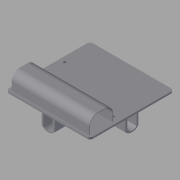
# Autodesk Inventor part: finalbody
Saved by Autodesk Inventor 2015 (Build 190159000, 159)
## iProperties
Created: 2015-11-09
Part Number: finalbody
Material: Generic
Document SubType Name: Modeling
Designer: Ross
Density: 1 g/cm^3
Appearance: Default
Author: Ross
Autodesk Inventor part; units mm, degrees
ref_plane "YZ Plane" through (0, 0, 0) normal (1, 0, 0) x (0, 1, 0)
ref_plane "XZ Plane" through (0, 0, 0) normal (0, 1, 0) x (-1, 0, 0)
sketch "Sketch1" plane through (0, 0, 0) normal (0, 1, 0) x (-1, 0, 0)
  line L0 (70, 0) -> (70, -70)
  line L1 (70, -70) -> (0, -70)
  line L2 (-70, 0) -> (-70, 70)
  line L3 (-70, 70) -> (0, 70)
  line L4 (0, 70) -> (70, 70)
  line L5 (70, 70) -> (70, 0)
  line L6 (0, -70) -> (-70, -70)
  line L7 (-70, -70) -> (-70, 0)
  point P0 (0, 0)
  constraints: 16 end point, 4 perpendicular, 2 point on line, 1 vertical
extrude "Extrusion1" add sketch "Sketch1" along normal blind 3
fillet "Fillet1" radius 5 3 edges at (70, 1.5, 70) (70, 1.5, -70) (-70, 1.5, 70)
fillet "Fillet2" radius 5 1 edges at (-70, 1.5, -70)
ref_plane "Work Plane1" through (65, 0, 65) normal (1, 0, 0) x (0, 0, -1)
sketch "Sketch5" plane through (65, 0, 65) normal (1, 0, 0) x (0, 0, -1)
  line L0 (0, 3) -> (0, 15.5)
  arc A0 (12.5, 28) -> (0, 15.5) centre (12.5, 15.5) ccw
  line L1 (12.5, 28) -> (25, 28)
  arc A1 (37.5, 15.5) -> (25, 28) centre (25, 15.5) ccw
  line L2 (37.5, 15.5) -> (37.5, 3)
  line L3 (0, 3) -> (130, 3) projected
  line L4 (0, 3) -> (-1, 3)
  line L5 (-5, 3) -> (0, 3) projected
  line L6 (-1, 3) -> (-1, 15.5)
  arc A2 (12.5, 29) -> (-1, 15.5) centre (12.5, 15.5) ccw
  line L7 (12.5, 29) -> (25, 29)
  arc A3 (38.5, 15.5) -> (25, 29) centre (25, 15.5) ccw
  line L8 (38.5, 15.5) -> (38.5, 3)
  line L9 (38.5, 3) -> (37.5, 3)
  line L10 (0, 3) -> (-1, 3)
  line L11 (0, 0) -> (0, 3) projected
  point P0 (65, 0)
  dimension "d9" = 12.5
  dimension "d11" = 12.5
  dimension "d12" = 1
  constraints: 18 end point, 8 point on circle, 4 centre point, 3 perpendicular, 3 point on line, 2 coincident, 2 vertical, 1 collinear, 1 horizontal, 1 parallel
  measures "d9" distance of L0.start L0.end
  measures "d11" distance of L1.start L1.end
  measures "d12" distance of L0.start L4.end
extrude "Extrusion2" add sketch "Sketch5" against normal blind 130 contours L4 L6 A2 L7 A3 L8 L3 L2 A1 L1 A0 L0
sketch "Sketch6" plane through (70, 0, 65) normal (1, 0, 0) x (0, 0, -1)
  line L0 (65, 0) -> (57.2, 0)
  line L1 (130, 0) -> (0, 0) projected
  line L2 (65, 0) -> (72.8, 0)
  line L3 (57.2, 0) -> (57.2, -18)
  line L4 (72.8, 0) -> (72.8, -18)
  line L5 (65, 0) -> (65, -10)
  arc A0 (57.2, -18) -> (72.8, -18) centre (65, -10.2437) ccw
  line L6 (57.2, 0) -> (54.2, 0)
  line L7 (54.2, 0) -> (54.2, -18)
  line L8 (72.8, 0) -> (75.8, 0)
  line L9 (75.8, 0) -> (75.8, -18)
  arc A1 (54.2, -18) -> (75.8, -18) centre (65, -9.0916) ccw
  dimension "d17" = 18
  dimension "d21" = 3
  dimension "d22" = 3
  constraints: 18 end point, 4 point on circle, 4 point on line, 3 perpendicular, 2 centre point, 2 vertical
  measures "d17" distance of L0.end L3.end
  measures "d21" distance of L0.end L6.end
  measures "d22" distance of L2.end L8.end
extrude "Extrusion3" add sketch "Sketch6" against normal blind 18 contours L3 A0 L4 L1 L9 A1 L7
pattern_circular "Circular Pattern1" count 4 over 360 about axis through (0, -10, 0) along (0, 1, 0) of "Extrusion3"
sketch "Sketch8" plane through (0, 3, 0) normal (0, 1, 0) x (1, 0, 0)
  circle A0 centre (58.4636, -19.348) radius 2.5
  point P0 (0, 0)
  dimension "d35" = 5
  constraints: 1 centre point
  measures "d35" diameter of A0
extrude "Extrusion5" cut sketch "Sketch8" against normal blind 3
sketch "Sketch9" plane through (0, 3, 0) normal (0, 1, 0) x (1, 0, 0)
  circle A0 centre (-60.6489, 18.9578) radius 2.5
  point P0 (0, 0)
  dimension "d39" = 5
  constraints: 1 centre point
  measures "d39" diameter of A0
extrude "Extrusion6" cut sketch "Sketch9" against normal blind 3
body "Solid1"
